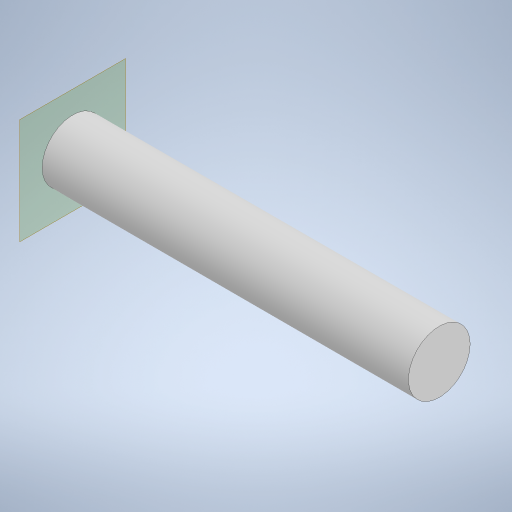
# Autodesk Inventor part: Piston Assembly Cast Image 1
Saved by Autodesk Inventor 2023 (Build 270158000, 158)
## iProperties
Created: 2022-12-28
Part Number: Piston Assembly Cast Image 1
Material: Generic
Document SubType Name: Modeling
Designer: tgr41
Density: 1 g/cm^3
Appearance: Default
Author: tgr41
Autodesk Inventor part; units mm, degrees
ref_plane "YZ Plane" through (0, 0, 0) normal (1, 0, 0) x (0, 1, 0)
ref_plane "XZ Plane" through (0, 0, 0) normal (0, 1, 0) x (-1, 0, 0)
ref_plane "XY Plane" through (0, 0, 0) normal (0, 0, 1) x (1, 0, 0)
ref_plane "Work Plane1" through (-12.7, 0, 0) normal (-1, 0, 0) x (0, 0, 1)
sketch "Sketch3" plane through (-12.7, 0, 0) normal (-1, 0, 0) x (0, 0, 1)
  circle A0 centre (0, 0) radius 6.35
  constraints: 1 centre point, 1 coincident
extrude "Extrusion2" add sketch "Sketch3" against normal blind 76.2
draft "FaceDraft1" angle 0.05 pull direction (-1, 0, 0) faces at (38.1, -1.0186, 6.2678) fixed edges at (-12.7, 0, -6.35)
body "Solid2"
